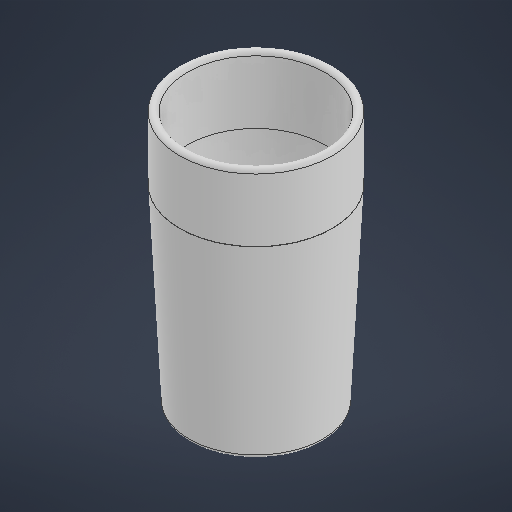
# Autodesk Inventor part: Coctelera
Saved by Autodesk Inventor 2026 (Build 300175050, 175E)
## iProperties
Created: 2025-12-08
Part Number: Coctelera
Material: Genérico
Document SubType Name: Modeling
Designer: David
Density: 1 g/cm^3
Appearance: Valor por defecto
Author: David
Autodesk Inventor part; units mm, degrees
ref_plane "YZ Plane" through (0, 0, 0) normal (1, 0, 0) x (0, 1, 0)
ref_plane "XZ Plane" through (0, 0, 0) normal (0, 1, 0) x (-1, 0, 0)
ref_plane "XY Plane" through (0, 0, 0) normal (0, 0, 1) x (1, 0, 0)
sketch "Boceto1" plane through (0, 0, 0) normal (0, 0, 1) x (1, 0, 0)
  line L0 (0, 0) -> (35, 0)
  line L1 (40, 100) -> (35, 0)
  line L2 (40, 100) -> (40, 135)
  line L3 (40, 135) -> (0, 135)
  line L4 (0, 135) -> (0, 0)
  dimension "d0" = 35
  constraints: 10 end point, 2 perpendicular, 1 horizontal
  measures "d0" distance of L0.start L0.end
sketch "Boceto2" plane through (0, 0, 0) normal (0, 0, 1) x (1, 0, 0)
  point P0 (0, 0)
revolve "Revolución1" add sketch "Boceto1" angle 360 about axis through (0, 135, 0) along (0, -1, 0)
fillet "Empalme1" radius 2 1 edges at (-35, 0, 0)
fillet "Empalme2" radius 2 1 edges at (-40, 135, 0)
fillet "Empalme3" radius 2 1 edges at (-40, 100, 0)
sketch "Boceto3" plane through (0, 135, 0) normal (0, 1, 0) x (1, 0, 0)
  circle A0 centre (0, 0) radius 32.5
  dimension "d8" = 65
  constraints: 1 centre point, 1 coincident
  measures "d8" diameter of A0
extrude "Extrusión1" cut sketch "Boceto3" against normal blind 125
sketch "Boceto4" plane through (0, 135, 0) normal (0, 1, 0) x (1, 0, 0)
  circle A0 centre (0, 0) radius 36
  dimension "d11" = 72
  constraints: 1 centre point, 1 coincident
  measures "d11" diameter of A0
extrude "Extrusión2" cut sketch "Boceto4" against normal blind 35
fillet "Empalme4" radius 2 1 edges at (-36, 135, 0)
fillet "Empalme5" radius 1981.5 1 edges at (-32.5, 100, 0)
